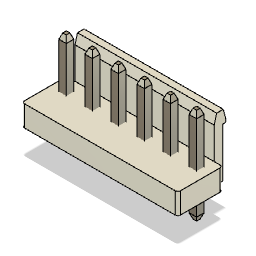
B6P-VH (Autodesk Fusion 360 design; units mm, degrees)
Autodesk Fusion 360 part; units mm, degrees
sketch "Skizze1" plane through (0, 0, 0) normal (0, 1, 0) x (1, 0, 0)
  line L0 (-11.85, 3.4) -> (11.85, 3.4)
  line L1 (11.85, 3.4) -> (11.85, -3.4)
  line L2 (11.85, -3.4) -> (-11.85, -3.4)
  line L3 (-11.85, -3.4) -> (-11.85, 3.4)
  line L4 (0, 3.4) -> (0, -3.4) construction
  dimension "d9" = 23.7
  dimension "d10" = 6.8
  constraint horizontal L0
  constraint vertical L1
  constraint horizontal L2
  constraint vertical L3
  constraint midpoint L0 L4.start
  constraint midpoint L2 L4.end
  constraint midpoint L4 origin
  measures "d9" distance of L0.start L0.end
  measures "d10" distance of L0.start L2.end
extrude "Extrusion1" add sketch "Skizze1" along normal blind 3.2 makes body 1
sketch "Skizze3" plane through (0, 0, 0) normal (1, 0, 0) x (0, 0, -1)
  line L0 (3.4, 0) -> (3.4, 3.2)
  line L1 (3.4, 0) -> (4.7, 0)
  line L2 (4.7, 0) -> (4.7, 9.4)
  line L3 (4.7, 9.4) -> (3.4, 9.4) construction
  line L4 (3.4, 9.4) -> (3.4, 0)
  line L5 (4.7, 9.4) -> (5.15, 9.4)
  line L6 (5.15, 9.4) -> (5.15, 0)
  line L7 (5.15, 0) -> (4.7, 0)
  line L8 (4.7, 0) -> (4.7, 9.4) construction
  line L9 (3.4, 8.0005) -> (3.775, 9.4)
  line L10 (4.775, 9.4) -> (5.15, 8.0005)
  line L11 (5.15, 7.5005) -> (4.7, 7.5005)
  line L12 (4.775, 9.4) -> (3.775, 9.4)
  line L13 (3.775, 9.4) -> (4.775, 9.4) construction
  line L14 (4.775, 9.4) -> (5.15, 9.4) construction
  line L15 (3.775, 9.4) -> (3.4, 9.4) construction
  line L16 (5.15, 9.4) -> (4.775, 9.4) construction
  line L17 (5.15, 8.0005) -> (5.15, 7.5005) construction
  line L18 (5.15, 7.5005) -> (5.15, 8.0005) construction
  line L19 (5.15, 9.4) -> (3.4, 9.4)
  line L20 (5.15, 0) -> (3.4, 0)
  dimension "d31" = 9.4
  dimension "d33" = 1.3
  dimension "d35" = 90
  dimension "d36" = 75
  dimension "d37" = 75
  dimension "d39" = 1
  dimension "d42" = 0.5
  dimension "d48" = 1.75
  constraint horizontal L1
  constraint vertical L2
  constraint horizontal L3
  constraint vertical L4
  constraint coincident L0.start L1.start
  constraint horizontal L5
  constraint vertical L6
  constraint horizontal L7
  constraint vertical L8
  constraint coincident L4 L9.start
  constraint coincident L3 L9.end
  constraint coincident L3 L10.start
  constraint coincident L6 L10.end
  constraint coincident L6 L11.start
  constraint coincident L2 L11.end
  constraint equal L15 L16
  constraint coincident L1.end L2.start
  measures "d31" distance of L1.end L2.end
  measures "d33" distance of L0.start L1.end
  measures "d35" angle of L6 L11
  measures "d36" angle of L3 L10
  measures "d37" angle of L3 L9
  measures "d39" distance of L9.end L10.start
  measures "d42" distance of L10.end L11.start
  measures "d48" distance of L6.end L0.start
sketch "Skizze2" plane through (0, 0, 0) normal (0, 1, 0) x (1, 0, 0)
  line L0 (-9.33, 0.83) -> (-10.47, 0.83)
  line L1 (-10.47, 0.83) -> (-10.47, 1.97)
  line L2 (-10.47, 1.97) -> (-9.33, 1.97)
  line L3 (-9.33, 1.97) -> (-9.33, 0.83)
  line L4 (-11.85, 3.4) -> (11.85, 3.4)
  line L5 (11.85, 3.4) -> (11.85, -3.4)
  line L6 (11.85, -3.4) -> (-11.85, -3.4)
  line L7 (-11.85, -3.4) -> (-11.85, 3.4)
  line L8 (0, 3.4) -> (0, 1.4) construction
  line L9 (-9.33, 1.4) -> (-10.47, 1.4) construction
  line L10 (0, 1.4) -> (-9.9, 1.4)
  point P0 (-9.9, 1.4)
  dimension "d16" = 1.14
  dimension "d17" = 1.14
  dimension "d24" = 2
  dimension "d26" = 9.9
  constraint horizontal L0
  constraint vertical L1
  constraint horizontal L2
  constraint vertical L3
  constraint midpoint L4 L8.start
  constraint perpendicular L4 L8
  constraint midpoint L3 L9.start
  constraint midpoint L1 L9.end
  constraint midpoint L9 P0
  constraint horizontal L10
  constraint coincident P0 L10.end
  measures "d16" distance of L0.start L0.end
  measures "d17" distance of L0.start L2.end
  measures "d24" distance of L8.start L8.end
  measures "d26" distance of L8.end P0
extrude "Extrusion3" add sketch "Skizze3" along normal mid plane 21.16 contours L0 L1 L2 L4 L9 L12 L19 L20 | L2 L5 L6 L10 L11 L12 L19 bodies 1
extrude "Extrusion2" add sketch "Skizze2" along normal blind 10.9 and the other way blind 3.7 separate body contours L0 L1 L2 L3 makes body 2
chamfer "Fase2" distance 0.3 angle 70 8 edges at (-9.9, 10.9, -0.83) (-9.33, 10.9, -1.4) (-9.9, 10.9, -1.97) (-10.47, 10.9, -1.4) (-9.33, -3.7, -1.4) (-9.9, -3.7, -0.83) (-10.47, -3.7, -1.4) (-9.9, -3.7, -1.97) measured on face at (-9.71, 10.9, -1.21) measured on face at (-9.71, 10.9, -1.21) measured on face at (-9.71, 10.9, -1.21) measured on face at (-9.71, 10.9, -1.21) measured on face at (-9.71, -3.7, -1.21) measured on face at (-9.71, -3.7, -1.21) measured on face at (-9.71, -3.7, -1.21) measured on face at (-9.71, -3.7, -1.21) on bodies 2
pattern_linear "R-Anordnung1" count 6 spacing 3.96 along (1, 0, 0) of bodies 2 makes body 3 at (-5.37, 1.4414, -1.59) makes body 4 at (-1.41, 1.4414, -1.59) makes body 5 at (2.55, 1.4414, -1.59) makes body 6 at (6.51, 1.4414, -1.59) makes body 7 at (10.47, 1.4414, -1.59)
fillet "Abrundung1" radius 0.4 4 edges at (11.85, 1.6, -3.4) (11.85, 1.6, 3.4) (-11.85, 1.6, 3.4) (-11.85, 1.6, -3.4) on bodies 1
equation "n = 6" comment "Number of pins"
equation "P = 3.96 mm" comment "Pin pitch"
equation "B1 = A1 + ( 1.95 mm * 2 )" comment "Width of bottom plate"
equation "A1 = ( n - 1 ) * P" comment "Total width of all pins"
equation "C1 = 6.8 mm" comment "Height of bottom plate"
equation "H1 = 9.4 mm" comment "Height of latching plate"
equation "O1 = 2 mm" comment "Vertical offset pin-center to bottom plate border"
equation "d9 = B1"
equation "d10 = C1"
equation "D1 = 3.2 mm" comment "Total depth of bottom plate"
equation "Pw = 1.14 mm" comment "Width & height of square pin"
equation "d13 = D1"
equation "d16 = Pw"
equation "d17 = Pw"
equation "LPinTop = 7.7 mm + D1" comment "Length of the pin measured from the bottom plane to the top of the pin (away from PCB)"
equation "LPinBottom = 14.6 mm - LPinTop" comment "Length of the pin in bottom direction, measured from the bottom plane"
equation "d20 = LPinTop"
equation "d22 = LPinBottom"
equation "d24 = O1"
equation "Pin1XOffset = ( ( n - 1 ) * P ) / 2" comment "First pin X offset measured from the X axis"
equation "d26 = Pin1XOffset"
equation "d27 = n"
equation "d29 = P"
equation "d31 = H1"
equation "D2 = 1.3 mm" comment "(Measured) depth of latching plate (narrowest section)"
equation "d33 = D2"
equation "d35 = alpha"
equation "d36 = 90 deg - beta"
equation "d37 = 90 deg - beta"
equation "Wx1 = 1.0 mm" comment "(Measured) Width of the topmost part of the latching plate"
equation "Hx1 = 0.5 mm" comment "(Measured) Height of the latching surface facing away from the pins"
equation "alpha = 90 deg" comment "Angle of the latching surface. Shown by the datasheet as ~45°but real parts have 90°"
equation "d42 = Hx1"
equation "beta = 15 deg" comment "(Estimated) Latching plate tapering angle"
equation "WL1 = 1.27 mm" comment "(Measured) With of the section of the bottom plate where there is no latching plate per side)"
equation "d45 = B1 - ( WL1 * 2 )"
equation "Dlatch = 1.75 mm" comment "(Measured) Total depth of latching plate"
equation "d48 = Dlatch"
equation "d54 = delta"
equation "delta = 70 deg" comment "(Estimated) Taper angle of the pin top & bottoms"
named bodies: "Bottom plate", "Pin", "Pin1 (1)", "Pin (1)", "Pin (2)", "Pin (3)", "Pin (4)"
